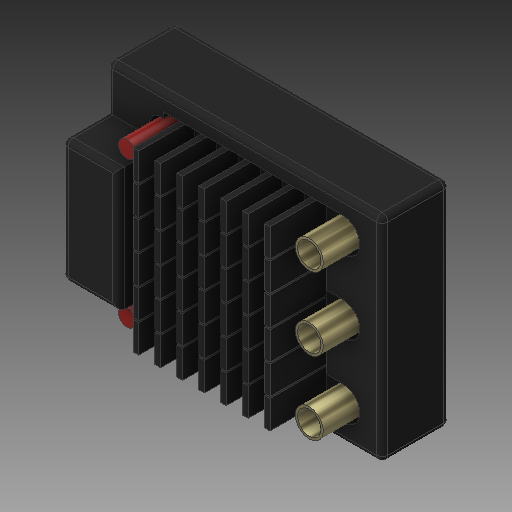
# Autodesk Inventor part: サイドワインダーV3
Saved by Autodesk Inventor 2019 (Build 230136000, 136)
## iProperties
Part Number: サイドワインダーV3
Material: 一般
Document SubType Name: Modeling
Designer: 雪村
Density: 1.83447 g/cm^3
Appearance: ゴム - 黒
Mass: 55.5 g
Surface Area: 148.747 cm^2
Volume: 30.254 cm^3
Author: 雪村
Autodesk Inventor part; units mm, degrees
ref_plane "YZ Plane" through (0, 0, 0) normal (1, 0, 0) x (0, 1, 0)
ref_plane "XZ Plane" through (0, 0, 0) normal (0, 1, 0) x (-1, 0, 0)
ref_plane "XY Plane" through (0, 0, 0) normal (0, 0, 1) x (1, 0, 0)
sketch "スケッチ1" plane through (0, 0, 0) normal (0, 0, 1) x (1, 0, 0)
  line L0 (0, 0) -> (49, 0)
  line L1 (49, 0) -> (49, 38)
  line L2 (49, 38) -> (0, 38)
  line L3 (0, 38) -> (0, 0)
  dimension "d0" = 49
  dimension "d1" = 38
  constraints: 8 end point
  measures "d0" distance of L2.end L1.end
  measures "d1" distance of L1.end L0.end
extrude "押し出し1" add sketch "スケッチ1" along normal blind 12
sketch "スケッチ2" plane through (0, 0, 12) normal (0, 0, 1) x (1, 0, 0)
  line L0 (10, 35) -> (39, 35)
  line L1 (39, 35) -> (39, 3)
  line L2 (39, 3) -> (10, 3)
  line L3 (10, 3) -> (10, 35)
  line L4 (0, 0) -> (49, 0) projected
  line L5 (49, 0) -> (49, 38) projected
  line L6 (49, 38) -> (0, 38) projected
  line L7 (0, 38) -> (0, 0) projected
  dimension "d5" = 3
  dimension "d6" = 3
  dimension "d7" = 10
  dimension "d8" = 10
  constraints: 8 end point, 2 horizontal, 2 vertical
  measures "d5" distance between parallel lines of L6 L0
  measures "d6" distance between parallel lines of L4 L2
  measures "d7" distance between parallel lines of L3 L7
  measures "d8" distance between parallel lines of L5 L1
extrude "押し出し2" cut sketch "スケッチ2" against normal blind 2 contours L0 L1 L2 L3
sketch "スケッチ3" plane through (0, 0, 12) normal (0, 0, 1) x (1, 0, 0)
  line L0 (10, 3) -> (10, 35) projected
  line L1 (10, 35) -> (39, 35) projected
  line L2 (39, 35) -> (39, 3) projected
  line L3 (39, 3) -> (10, 3) projected
  line L4 (0, 0) -> (49, 0) projected
  line L5 (49, 0) -> (49, 38) projected
  line L6 (49, 38) -> (0, 38) projected
  line L7 (0, 38) -> (0, 0) projected
  line L8 (10, 3) -> (10, 35) projected
  line L9 (0, 30) -> (10, 30)
  line L10 (10, 30) -> (10, 8)
  line L11 (10, 8) -> (0, 8)
  line L12 (0, 8) -> (0, 30)
  dimension "d11" = 8
  dimension "d12" = 8
  constraints: 8 end point, 2 horizontal, 2 point on line, 2 vertical
  measures "d11" distance between parallel lines of L9 L6
  measures "d12" distance between parallel lines of L4 L11
extrude "押し出し3" add sketch "スケッチ3" along normal blind 8 contours L11 L7 L9 L0
sketch "スケッチ4" plane through (0, 0, 12) normal (0, 0, 1) x (1, 0, 0)
  line L0 (0, 30) -> (10, 30) projected
  line L1 (10, 30) -> (10, 35) projected
  line L2 (10, 3) -> (10, 8) projected
  line L3 (10, 8) -> (0, 8) projected
  line L4 (0, 8) -> (0, 0) projected
  line L5 (0, 0) -> (49, 0) projected
  line L6 (49, 0) -> (49, 38) projected
  circle A0 centre (9.5, 32) radius 2
  circle A1 centre (9.5, 6) radius 2
  line L7 (10, 8) -> (0, 8) projected
  line L8 (0, 30) -> (10, 30) projected
  arc A2 (42, 29) -> (42, 35) centre (42, 32) ccw
  arc A3 (42, 16) -> (42, 22) centre (42, 19) ccw
  arc A4 (42, 3) -> (42, 9) centre (42, 6) ccw
  line L9 (39, 35) -> (39, 3) projected
  line L10 (39, 3) -> (10, 3) projected
  line L11 (39, 35) -> (42, 35)
  line L12 (42, 29) -> (39, 29)
  line L13 (42, 9) -> (39, 9)
  line L14 (39, 35) -> (39, 3) projected
  line L15 (42, 3) -> (39, 3)
  line L16 (42, 16) -> (39, 16)
  line L17 (42, 22) -> (39, 22)
  line L18 (39, 35) -> (39, 29)
  line L19 (39, 22) -> (39, 16)
  line L20 (39, 9) -> (39, 3)
  point P0 (0, 38)
  dimension "d15" = 4
  dimension "d16" = 4
  dimension "d17" = 0.5
  dimension "d18" = 0.5
  dimension "d19" = 6
  dimension "d20" = 6
  dimension "d21" = 6
  dimension "d22" = 13
  dimension "d23" = 13
  constraints: 18 end point, 10 tangent, 6 horizontal, 6 point on circle, 5 centre point, 4 point on line
  measures "d15" diameter of A0
  measures "d16" diameter of A1
  measures "d17" distance from line of L1 A0.centre
  measures "d18" distance from line of L2 A1.centre
  measures "d19" diameter of A2
  measures "d20" diameter of A3
  measures "d21" diameter of A4
  measures "d22" distance of A3.centre A2.centre
  measures "d23" distance of A4.centre A3.centre
extrude "押し出し5" cut sketch "スケッチ4" against normal blind 2 contours A0 L1 | A0 L1 | A1 L2 | L2 A1 | L9 L11 A2 L12 | L9 L17 A3 L16 | L9 L13 A4 L15
sketch "スケッチ5" plane through (0, 0, 10) normal (0, 0, 1) x (1, 0, 0)
  line L0 (10, 3) -> (10, 4.0635) projected
  line L1 (42, 3) -> (10, 3) projected
  arc A0 (42, 3) -> (42, 9) centre (42, 6) ccw projected
  line L2 (39, 9) -> (42, 9) projected
  line L3 (39, 16) -> (39, 9) projected
  line L4 (42, 16) -> (39, 16) projected
  arc A1 (42, 16) -> (42, 22) centre (42, 19) ccw projected
  line L5 (39, 22) -> (42, 22) projected
  line L6 (39, 29) -> (39, 22) projected
  line L7 (42, 29) -> (39, 29) projected
  arc A2 (42, 29) -> (42, 35) centre (42, 32) ccw projected
  line L8 (10, 35) -> (42, 35) projected
  line L9 (10, 33.9365) -> (10, 35) projected
  arc A3 (10, 33.9365) -> (10, 30.0635) centre (9.5, 32) ccw projected
  line L10 (10, 7.9365) -> (10, 30.0635) projected
  arc A4 (10, 7.9365) -> (10, 4.0635) centre (9.5, 6) ccw projected
  circle A5 centre (42, 32) radius 2.5
  circle A6 centre (42, 19) radius 2.5
  circle A7 centre (42, 6) radius 2.5
  circle A8 centre (9.5, 32) radius 1.5
  circle A9 centre (9.5, 6) radius 1.5
  point P0 (0, 0)
  dimension "d28" = 5
  dimension "d29" = 5
  dimension "d30" = 5
  dimension "d31" = 3
  dimension "d32" = 3
  constraints: 5 centre point, 5 coincident
  measures "d28" diameter of A5
  measures "d29" diameter of A6
  measures "d30" diameter of A7
  measures "d31" diameter of A8
  measures "d32" diameter of A9
extrude "押し出し6" add sketch "スケッチ5" along normal blind 8 contours A5 | A6 | A7 | A8 | A9
sketch "スケッチ6" plane through (42, 32, 18) normal (0, 0, 1) x (1, 0, 0)
  circle A0 centre (0, 0) radius 2.5 projected
  circle A1 centre (0, -13) radius 2.5 projected
  circle A2 centre (0, -26) radius 2.5 projected
  circle A3 centre (0, 0) radius 2.1
  circle A4 centre (0, -13) radius 2.1
  circle A5 centre (0, -26) radius 2.1
  point P0 (-42, -32)
  dimension "d35" = 4.2
  dimension "d36" = 4.2
  dimension "d37" = 4.2
  constraints: 3 centre point, 3 coincident
  measures "d35" diameter of A3
  measures "d36" diameter of A4
  measures "d37" diameter of A5
extrude "押し出し7" cut sketch "スケッチ6" against normal blind 8 contours A3 | A4 | A5
sketch "スケッチ10" plane through (0, 0, 10) normal (0, 0, 1) x (1, 0, 0)
  circle A0 centre (42, 19) radius 2.5 projected
  circle A1 centre (9.5, 6) radius 1.5 projected
  circle A2 centre (9.5, 32) radius 1.5 projected
  circle A3 centre (42, 32) radius 2.5 projected
  circle A4 centre (42, 6) radius 2.5 projected
  line L0 (10, 3) -> (10, 4.0635) projected
  line L1 (42, 3) -> (10, 3) projected
  arc A5 (42, 3) -> (42, 9) centre (42, 6) ccw projected
  line L2 (39, 9) -> (42, 9) projected
  line L3 (39, 16) -> (39, 9) projected
  line L4 (42, 16) -> (39, 16) projected
  arc A6 (42, 16) -> (42, 22) centre (42, 19) ccw projected
  line L5 (39, 22) -> (42, 22) projected
  line L6 (39, 29) -> (39, 22) projected
  line L7 (42, 29) -> (39, 29) projected
  arc A7 (42, 29) -> (42, 35) centre (42, 32) ccw projected
  line L8 (10, 35) -> (42, 35) projected
  line L9 (10, 33.9365) -> (10, 35) projected
  arc A8 (10, 33.9365) -> (10, 30.0635) centre (9.5, 32) ccw projected
  line L10 (10, 7.9365) -> (10, 30.0635) projected
  arc A9 (10, 7.9365) -> (10, 4.0635) centre (9.5, 6) ccw projected
  line L11 (11.2, 34.75) -> (11.2, 3.25)
  line L12 (15, 34.75) -> (15, 3.25)
  line L13 (15.1, 34.75) -> (15.1, 3.25)
  line L14 (18.9, 34.75) -> (18.9, 3.25)
  line L15 (19, 34.75) -> (19, 3.25)
  line L16 (22.8, 3.25) -> (22.8, 34.75)
  line L17 (22.9, 34.75) -> (22.9, 3.25)
  line L18 (26.7, 3.25) -> (26.7, 34.75)
  line L19 (26.8, 34.75) -> (26.8, 3.25)
  line L20 (30.6, 3.25) -> (30.6, 34.75)
  line L21 (30.7, 34.75) -> (30.7, 3.25)
  line L22 (34.5, 3.25) -> (34.5, 34.75)
  line L23 (34.6, 34.75) -> (34.6, 3.25)
  line L24 (38.4, 3.25) -> (38.4, 34.75)
  line L25 (12.6, 34.75) -> (12.6, 29.75)
  line L26 (13.6, 29.75) -> (13.6, 34.75)
  line L27 (12.6, 29.75) -> (13.6, 29.75)
  line L28 (12.6, 29.45) -> (13.6, 29.45)
  line L29 (13.6, 24.45) -> (13.6, 29.45)
  line L30 (12.6, 24.15) -> (13.6, 24.15)
  line L31 (13.6, 19.15) -> (13.6, 24.15)
  line L32 (12.6, 18.85) -> (13.6, 18.85)
  line L33 (12.6, 19.15) -> (13.6, 19.15)
  line L34 (12.6, 18.85) -> (12.6, 13.85)
  line L35 (13.6, 13.55) -> (12.6, 13.55)
  line L36 (12.6, 13.85) -> (13.6, 13.85)
  line L37 (13.6, 13.85) -> (13.6, 18.85)
  line L38 (12.6, 29.45) -> (12.6, 24.45)
  line L39 (12.6, 24.15) -> (12.6, 19.15)
  line L40 (12.6, 24.45) -> (13.6, 24.45)
  line L41 (12.6, 13.55) -> (12.6, 8.55)
  line L42 (12.6, 8.25) -> (12.6, 3.25)
  line L43 (13.6, 3.25) -> (13.6, 8.25)
  line L44 (13.6, 8.55) -> (13.6, 13.55)
  line L45 (12.6, 8.55) -> (13.6, 8.55)
  line L46 (13.6, 8.25) -> (12.6, 8.25)
  line L47 (12.6, 3.25) -> (13.6, 3.25)
  line L48 (16.5, 3.25) -> (17.5, 3.25)
  line L49 (17.5, 3.25) -> (17.5, 8.25)
  line L50 (15, 8.55) -> (15.1, 8.55)
  line L51 (16.5, 8.55) -> (17.5, 8.55)
  line L52 (17.5, 8.25) -> (16.5, 8.25)
  line L53 (15.1, 8.25) -> (15, 8.25)
  line L54 (16.5, 8.25) -> (16.5, 3.25)
  line L55 (15, 13.85) -> (15.1, 13.85)
  line L56 (15.1, 13.55) -> (15, 13.55)
  line L57 (16.5, 13.55) -> (16.5, 8.55)
  line L58 (17.5, 8.55) -> (17.5, 13.55)
  line L59 (16.5, 13.85) -> (17.5, 13.85)
  line L60 (17.5, 13.55) -> (16.5, 13.55)
  line L61 (17.5, 13.85) -> (17.5, 18.85)
  line L62 (16.5, 18.85) -> (16.5, 13.85)
  line L63 (15, 19.15) -> (15.1, 19.15)
  line L64 (16.5, 19.15) -> (17.5, 19.15)
  line L65 (15, 18.85) -> (15.1, 18.85)
  line L66 (16.5, 18.85) -> (17.5, 18.85)
  line L67 (15, 24.45) -> (15.1, 24.45)
  line L68 (15, 24.15) -> (15.1, 24.15)
  line L69 (16.5, 24.15) -> (16.5, 19.15)
  line L70 (17.5, 19.15) -> (17.5, 24.15)
  line L71 (16.5, 24.15) -> (17.5, 24.15)
  line L72 (16.5, 24.45) -> (17.5, 24.45)
  line L73 (15, 29.75) -> (15.1, 29.75)
  line L74 (15, 29.45) -> (15.1, 29.45)
  line L75 (16.5, 34.75) -> (16.5, 29.75)
  line L76 (16.5, 29.45) -> (16.5, 24.45)
  line L77 (17.5, 24.45) -> (17.5, 29.45)
  line L78 (17.5, 29.75) -> (17.5, 34.75)
  line L79 (16.5, 29.75) -> (17.5, 29.75)
  line L80 (16.5, 29.45) -> (17.5, 29.45)
  line L81 (11.2, 34.75) -> (15.1, 34.75)
  line L82 (16.5, 34.75) -> (17.5, 34.75)
  line L83 (18.9, 34.75) -> (19, 34.75)
  line L84 (20.4, 34.75) -> (21.4, 34.75)
  line L85 (18.9, 29.75) -> (19, 29.75)
  line L86 (18.9, 29.45) -> (19, 29.45)
  line L87 (20.4, 34.75) -> (20.4, 29.75)
  line L88 (21.4, 29.75) -> (21.4, 34.75)
  line L89 (20.4, 29.75) -> (21.4, 29.75)
  line L90 (20.4, 29.45) -> (21.4, 29.45)
  line L91 (18.9, 24.45) -> (19, 24.45)
  line L92 (18.9, 24.15) -> (19, 24.15)
  line L93 (20.4, 29.45) -> (20.4, 24.45)
  line L94 (21.4, 24.45) -> (21.4, 29.45)
  line L95 (20.4, 24.15) -> (21.4, 24.15)
  line L96 (20.4, 24.45) -> (21.4, 24.45)
  line L97 (18.9, 18.85) -> (19, 18.85)
  line L98 (18.9, 19.15) -> (19, 19.15)
  line L99 (20.4, 24.15) -> (20.4, 19.15)
  line L100 (21.4, 19.15) -> (21.4, 24.15)
  line L101 (20.4, 19.15) -> (21.4, 19.15)
  line L102 (20.4, 18.85) -> (21.4, 18.85)
  line L103 (18.9, 13.85) -> (19, 13.85)
  line L104 (19, 13.55) -> (18.9, 13.55)
  line L105 (20.4, 18.85) -> (20.4, 13.85)
  line L106 (21.4, 13.85) -> (21.4, 18.85)
  line L107 (20.4, 13.85) -> (21.4, 13.85)
  line L108 (21.4, 13.55) -> (20.4, 13.55)
  line L109 (18.9, 8.55) -> (19, 8.55)
  line L110 (19, 8.25) -> (18.9, 8.25)
  line L111 (20.4, 13.55) -> (20.4, 8.55)
  line L112 (20.4, 8.25) -> (20.4, 3.25)
  line L113 (21.4, 3.25) -> (21.4, 8.25)
  line L114 (21.4, 8.55) -> (21.4, 13.55)
  line L115 (20.4, 8.55) -> (21.4, 8.55)
  line L116 (21.4, 8.25) -> (20.4, 8.25)
  line L117 (18.9, 3.25) -> (19, 3.25)
  line L118 (20.4, 3.25) -> (21.4, 3.25)
  line L119 (22.8, 3.25) -> (22.9, 3.25)
  line L120 (24.3, 3.25) -> (25.3, 3.25)
  line L121 (25.3, 3.25) -> (25.3, 8.25)
  line L122 (24.3, 8.25) -> (24.3, 3.25)
  line L123 (22.8, 8.55) -> (22.9, 8.55)
  line L124 (24.3, 8.55) -> (25.3, 8.55)
  line L125 (25.3, 8.25) -> (24.3, 8.25)
  line L126 (22.9, 8.25) -> (22.8, 8.25)
  line L127 (22.8, 13.85) -> (22.9, 13.85)
  line L128 (22.9, 13.55) -> (22.8, 13.55)
  line L129 (24.3, 13.55) -> (24.3, 8.55)
  line L130 (25.3, 8.55) -> (25.3, 13.55)
  line L131 (24.3, 13.85) -> (25.3, 13.85)
  line L132 (25.3, 13.55) -> (24.3, 13.55)
  line L133 (22.8, 19.15) -> (22.9, 19.15)
  line L134 (22.8, 18.85) -> (22.9, 18.85)
  line L135 (24.3, 18.85) -> (24.3, 13.85)
  line L136 (25.3, 13.85) -> (25.3, 18.85)
  line L137 (24.3, 19.15) -> (25.3, 19.15)
  line L138 (24.3, 18.85) -> (25.3, 18.85)
  line L139 (22.8, 24.45) -> (22.9, 24.45)
  line L140 (22.8, 24.15) -> (22.9, 24.15)
  line L141 (24.3, 24.15) -> (24.3, 19.15)
  line L142 (25.3, 19.15) -> (25.3, 24.15)
  line L143 (24.3, 24.45) -> (25.3, 24.45)
  line L144 (24.3, 24.15) -> (25.3, 24.15)
  line L145 (22.8, 29.45) -> (22.9, 29.45)
  line L146 (22.8, 29.75) -> (22.9, 29.75)
  line L147 (24.3, 34.75) -> (24.3, 29.75)
  line L148 (24.3, 29.45) -> (24.3, 24.45)
  line L149 (25.3, 24.45) -> (25.3, 29.45)
  line L150 (25.3, 29.75) -> (25.3, 34.75)
  line L151 (24.3, 29.75) -> (25.3, 29.75)
  line L152 (24.3, 29.45) -> (25.3, 29.45)
  line L153 (22.8, 34.75) -> (22.9, 34.75)
  line L154 (24.3, 34.75) -> (25.3, 34.75)
  line L155 (26.7, 34.75) -> (26.8, 34.75)
  line L156 (28.2, 34.75) -> (29.2, 34.75)
  line L157 (26.7, 29.75) -> (26.8, 29.75)
  line L158 (26.7, 29.45) -> (26.8, 29.45)
  line L159 (28.2, 34.75) -> (28.2, 29.75)
  line L160 (29.2, 29.75) -> (29.2, 34.75)
  line L161 (28.2, 29.75) -> (29.2, 29.75)
  line L162 (28.2, 29.45) -> (29.2, 29.45)
  line L163 (26.7, 24.45) -> (26.8, 24.45)
  line L164 (26.7, 24.15) -> (26.8, 24.15)
  line L165 (28.2, 29.45) -> (28.2, 24.45)
  line L166 (29.2, 24.45) -> (29.2, 29.45)
  line L167 (28.2, 24.45) -> (29.2, 24.45)
  line L168 (28.2, 24.15) -> (29.2, 24.15)
  line L169 (26.7, 19.15) -> (26.8, 19.15)
  line L170 (26.7, 18.85) -> (26.8, 18.85)
  line L171 (28.2, 24.15) -> (28.2, 19.15)
  line L172 (29.2, 19.15) -> (29.2, 24.15)
  line L173 (28.2, 19.15) -> (29.2, 19.15)
  line L174 (28.2, 18.85) -> (29.2, 18.85)
  line L175 (26.8, 13.55) -> (26.7, 13.55)
  line L176 (26.7, 13.85) -> (26.8, 13.85)
  line L177 (26.8, 8.25) -> (26.7, 8.25)
  line L178 (26.7, 8.55) -> (26.8, 8.55)
  line L179 (28.2, 13.85) -> (29.2, 13.85)
  line L180 (29.2, 13.55) -> (28.2, 13.55)
  line L181 (28.2, 8.55) -> (29.2, 8.55)
  line L182 (29.2, 8.25) -> (28.2, 8.25)
  line L183 (28.2, 18.85) -> (28.2, 13.85)
  line L184 (29.2, 13.85) -> (29.2, 18.85)
  line L185 (29.2, 3.25) -> (29.2, 8.25)
  line L186 (29.2, 8.55) -> (29.2, 13.55)
  line L187 (28.2, 13.55) -> (28.2, 8.55)
  line L188 (28.2, 8.25) -> (28.2, 3.25)
  line L189 (26.7, 3.25) -> (26.8, 3.25)
  line L190 (28.2, 3.25) -> (29.2, 3.25)
  line L191 (30.6, 3.25) -> (30.7, 3.25)
  line L192 (32.1, 3.25) -> (33.1, 3.25)
  line L193 (33.1, 3.25) -> (33.1, 8.25)
  line L194 (32.1, 8.25) -> (32.1, 3.25)
  line L195 (30.6, 8.55) -> (30.7, 8.55)
  line L196 (32.1, 8.55) -> (33.1, 8.55)
  line L197 (33.1, 8.25) -> (32.1, 8.25)
  line L198 (30.7, 8.25) -> (30.6, 8.25)
  line L199 (30.7, 13.55) -> (30.6, 13.55)
  line L200 (30.6, 13.85) -> (30.7, 13.85)
  line L201 (32.1, 13.85) -> (33.1, 13.85)
  line L202 (33.1, 13.55) -> (32.1, 13.55)
  line L203 (33.1, 8.55) -> (33.1, 13.55)
  line L204 (32.1, 13.55) -> (32.1, 8.55)
  line L205 (30.6, 18.85) -> (30.7, 18.85)
  line L206 (30.6, 19.15) -> (30.7, 19.15)
  line L207 (32.1, 19.15) -> (33.1, 19.15)
  line L208 (32.1, 18.85) -> (33.1, 18.85)
  line L209 (32.1, 18.85) -> (32.1, 13.85)
  line L210 (33.1, 13.85) -> (33.1, 18.85)
  line L211 (30.6, 24.45) -> (30.7, 24.45)
  line L212 (30.6, 24.15) -> (30.7, 24.15)
  line L213 (32.1, 24.45) -> (33.1, 24.45)
  line L214 (32.1, 24.15) -> (33.1, 24.15)
  line L215 (32.1, 24.15) -> (32.1, 19.15)
  line L216 (33.1, 19.15) -> (33.1, 24.15)
  line L217 (30.6, 29.45) -> (30.7, 29.45)
  line L218 (30.6, 29.75) -> (30.7, 29.75)
  line L219 (32.1, 29.75) -> (33.1, 29.75)
  line L220 (32.1, 29.45) -> (33.1, 29.45)
  line L221 (32.1, 34.75) -> (32.1, 29.75)
  line L222 (32.1, 29.45) -> (32.1, 24.45)
  line L223 (33.1, 24.45) -> (33.1, 29.45)
  line L224 (33.1, 29.75) -> (33.1, 34.75)
  line L225 (30.6, 34.75) -> (30.7, 34.75)
  line L226 (32.1, 34.75) -> (33.1, 34.75)
  line L227 (34.5, 34.75) -> (34.6, 34.75)
  line L228 (36, 34.75) -> (37, 34.75)
  line L229 (37, 29.75) -> (37, 34.75)
  line L230 (36, 34.75) -> (36, 29.75)
  line L231 (34.5, 29.45) -> (34.6, 29.45)
  line L232 (36, 29.45) -> (37, 29.45)
  line L233 (34.5, 29.75) -> (34.6, 29.75)
  line L234 (36, 29.75) -> (37, 29.75)
  line L235 (34.5, 24.45) -> (34.6, 24.45)
  line L236 (36, 24.45) -> (37, 24.45)
  line L237 (34.5, 24.15) -> (34.6, 24.15)
  line L238 (36, 24.15) -> (37, 24.15)
  line L239 (36, 29.45) -> (36, 24.45)
  line L240 (37, 24.45) -> (37, 29.45)
  line L241 (34.5, 19.15) -> (34.6, 19.15)
  line L242 (36, 19.15) -> (37, 19.15)
  line L243 (34.5, 18.85) -> (34.6, 18.85)
  line L244 (36, 18.85) -> (37, 18.85)
  line L245 (36, 24.15) -> (36, 19.15)
  line L246 (37, 19.15) -> (37, 24.15)
  line L247 (34.5, 13.85) -> (34.6, 13.85)
  line L248 (36, 13.85) -> (37, 13.85)
  line L249 (37, 13.55) -> (36, 13.55)
  line L250 (34.6, 13.55) -> (34.5, 13.55)
  line L251 (36, 18.85) -> (36, 13.85)
  line L252 (37, 13.85) -> (37, 18.85)
  line L253 (34.5, 8.55) -> (34.6, 8.55)
  line L254 (36, 8.55) -> (37, 8.55)
  line L255 (37, 8.25) -> (36, 8.25)
  line L256 (34.6, 8.25) -> (34.5, 8.25)
  line L257 (36, 13.55) -> (36, 8.55)
  line L258 (36, 8.25) -> (36, 3.25)
  line L259 (37, 3.25) -> (37, 8.25)
  line L260 (37, 8.55) -> (37, 13.55)
  line L261 (34.5, 3.25) -> (34.6, 3.25)
  line L262 (36, 3.25) -> (37, 3.25)
  point P0 (0, 0)
  dimension "d167" = 0.1
  dimension "d168" = 3.8
  dimension "d169" = 3.8
  dimension "d170" = 3.8
  dimension "d171" = 0.1
  dimension "d172" = 0.1
  dimension "d173" = 3.8
  dimension "d174" = 3.8
  dimension "d175" = 0.1
  dimension "d176" = 0.1
  dimension "d177" = 0.1
  dimension "d163" = 0.25
  dimension "d164" = 0.25
  dimension "d165" = 1.2
  dimension "d166" = 3.8
  dimension "d178" = 3.8
  constraints: 480 end point, 141 horizontal, 86 vertical, 3 point on line, 156 other
  measures "d163" distance from line of L8 L11.start
  measures "d164" distance from line of L1 L11.end
  measures "d165" distance between parallel lines of L11 L10
extrude "押し出し11" add sketch "スケッチ10" along normal blind 10 contours L26 L27 L25 L81 | L28 L29 L40 L38 | L30 L31 L33 L39 | L32 L37 L36 L34 | L44 L45 L41 L35 | L46 L43 L47 L42 | L54 L52 L49 L48 | L57 L60 L58 L51 | L62 L66 L61 L59 | L69 L71 L70 L64 | L76 L80 L77 L72 | L82 L78 L79 L75 | L84 L88 L89 L87 | L90 L94 L96 L93 | L95 L100 L101 L99 | L102 L106 L107 L105 | L114 L115 L111 L108 | L116 L113 L118 L112 | L122 L125 L121 L120 | L129 L132 L130 L124 | L135 L138 L136 L131 | L141 L144 L142 L137 | L148 L152 L149 L143 | L154 L150 L151 L147 | L156 L160 L161 L159 | L162 L166 L167 L165 | L168 L172 L173 L171 | L174 L184 L179 L183 | L186 L181 L187 L180 | L185 L190 L188 L182 | L194 L197 L193 L192 | L204 L202 L203 L196 | L209 L208 L210 L201 | L215 L214 L216 L207 | L222 L220 L223 L213 | L221 L226 L224 L219 | L228 L229 L234 L230 | L232 L240 L236 L239 | L238 L246 L242 L245 | L244 L252 L248 L251 | L260 L254 L257 L249 | L259 L262 L258 L255
fillet "フィレット1" radius 1 19 edges at (24.5, 0, 12) (24.5, 38, 12) (0, 4, 12) (0, 34, 12) (0, 19, 20) (5, 8, 20) (10, 19, 20) (5, 30, 20) (0, 8, 16) (0, 30, 16) (49, 19, 12) (49, 0, 6) (49, 38, 6) (49, 19, 0) (0, 0, 6) (24.5, 0, 0) (0, 19, 0) (0, 38, 6) (24.5, 38, 0)
